sgm (Autodesk Fusion 360 design; units mm, degrees)
Autodesk Fusion 360 part; units mm, degrees
(part 1 of 2)
sketch "Sketch3" plane through (0, 0, 0) normal (0, 1, 0) x (1, 0, 0)
  spline S0 degree 3 poles (81.8621, -52.3081) (79.4279, -54.4777) (76.4646, -57.15) (75.3004, -58.2613) knots 0 0 0 0 1 1 1 1
  spline S1 degree 3 poles (75.3004, -58.2613) (74.1098, -59.3725) (73.0779, -60.1927) (72.9721, -60.0869) knots 0 0 0 0 1 1 1 1
  spline S2 degree 3 poles (72.9721, -60.0869) (72.5223, -59.6635) (72.1783, -56.6208) (72.3106, -54.3454) knots 0 0 0 0 1 1 1 1
  spline S3 degree 3 poles (72.3106, -54.3454) (72.4958, -51.5673) (72.2313, -50.9323) (70.776, -50.6412) knots 0 0 0 0 1 1 1 1
  spline S4 degree 3 poles (70.776, -50.6412) (69.559, -50.4296) (68.7652, -50.9587) (67.8392, -52.5727) knots 0 0 0 0 1 1 1 1
  spline S5 degree 3 poles (67.8392, -52.5727) (67.4423, -53.2871) (65.9606, -55.7477) (64.5583, -58.076) knots 0 0 0 0 1 1 1 1
  spline S6 degree 3 poles (64.5583, -58.076) (60.6954, -64.3996) (60.3779, -64.9817) (60.034, -66.1194) knots 0 0 0 0 1 1 1 1
  spline S7 degree 3 poles (60.034, -66.1194) (59.6371, -67.4423) (60.0075, -67.9979) (61.2246, -67.9979) knots 0 0 0 0 1 1 1 1
  spline S8 degree 3 poles (61.2246, -67.9979) (62.3888, -67.9979) (63.0238, -67.2306) (64.0027, -64.7171) knots 0 0 0 0 1 1 1 1
  spline S9 degree 3 poles (64.0027, -64.7171) (64.6906, -62.9444) (67.019, -58.4465) (68.8446, -55.4302) knots 0 0 0 0 1 1 1 1
  line L0 (68.8446, -55.4302) -> (69.3208, -54.6365)
  line L1 (69.3208, -54.6365) -> (69.2944, -57.15)
  spline S10 degree 3 poles (69.2944, -57.15) (69.2944, -60.3779) (69.85, -62.8915) (70.776, -63.6852) knots 0 0 0 0 1 1 1 1
  spline S11 degree 3 poles (70.776, -63.6852) (71.4375, -64.2673) (71.5169, -64.2673) (72.2842, -63.8704) knots 0 0 0 0 1 1 1 1
  spline S12 degree 3 poles (72.2842, -63.8704) (72.734, -63.6323) (75.1946, -61.4892) (77.7346, -59.1079) knots 0 0 0 0 1 1 1 1
  spline S13 degree 3 poles (77.7346, -59.1079) (80.301, -56.7267) (82.4442, -54.8217) (82.4706, -54.8746) knots 0 0 0 0 1 1 1 1
  spline S14 degree 3 poles (82.4706, -54.8746) (82.5235, -54.901) (81.6769, -56.7796) (80.5921, -59.0285) knots 0 0 0 0 1 1 1 1
  spline S15 degree 3 poles (80.5921, -59.0285) (77.2848, -65.9342) (76.7556, -68.7652) (78.6077, -69.4002) knots 0 0 0 0 1 1 1 1
  spline S16 degree 3 poles (78.6077, -69.4002) (79.2163, -69.6119) (80.5921, -68.924) (81.1213, -68.1567) knots 0 0 0 0 1 1 1 1
  spline S17 degree 3 poles (81.1213, -68.1567) (81.5181, -67.5217) (81.5181, -67.4158) (81.1477, -66.9925) knots 0 0 0 0 1 1 1 1
  spline S18 degree 3 poles (81.1477, -66.9925) (80.7773, -66.5692) (80.7508, -66.3575) (81.0683, -65.1933) knots 0 0 0 0 1 1 1 1
  spline S19 degree 3 poles (81.0683, -65.1933) (81.5446, -63.3677) (82.2854, -61.4627) (83.7406, -58.2083) knots 0 0 0 0 1 1 1 1
  spline S20 degree 3 poles (83.7406, -58.2083) (84.4285, -56.7002) (85.2223, -54.7952) (85.5133, -53.975) knots 0 0 0 0 1 1 1 1
  spline S21 degree 3 poles (85.5133, -53.975) (85.8308, -53.1813) (86.4658, -51.8848) (86.9421, -51.1175) knots 0 0 0 0 1 1 1 1
  spline S22 degree 3 poles (86.9421, -51.1175) (87.4448, -50.3502) (87.8417, -49.6358) (87.8417, -49.5035) knots 0 0 0 0 1 1 1 1
  spline S23 degree 3 poles (87.8417, -49.5035) (87.8417, -49.2125) (86.9421, -48.4188) (86.5717, -48.4188) knots 0 0 0 0 1 1 1 1
  spline S24 degree 3 poles (86.5717, -48.4188) (86.4129, -48.4188) (84.2963, -50.165) (81.8621, -52.3081) knots 0 0 0 0 1 1 1 1
  spline S25 degree 3 poles (149.9658, -49.9269) (148.934, -51.0381) (146.6585, -54.7952) (145.124, -57.9967) knots 0 0 0 0 1 1 1 1
  spline S26 degree 3 poles (145.124, -57.9967) (143.6688, -61.0394) (142.8221, -61.9125) (139.356, -64.135) knots 0 0 0 0 1 1 1 1
  spline S27 degree 3 poles (139.356, -64.135) (137.2394, -65.5108) (135.9165, -65.9342) (135.3079, -65.5108) knots 0 0 0 0 1 1 1 1
  spline S28 degree 3 poles (135.3079, -65.5108) (134.8846, -65.1933) (134.8846, -65.0875) (135.3079, -63.7646) knots 0 0 0 0 1 1 1 1
  spline S29 degree 3 poles (135.3079, -63.7646) (136.0223, -61.5685) (137.9538, -57.8908) (140.3879, -54.0808) knots 0 0 0 0 1 1 1 1
  spline S30 degree 3 poles (140.3879, -54.0808) (141.605, -52.1494) (142.6104, -50.4031) (142.6104, -50.165) knots 0 0 0 0 1 1 1 1
  spline S31 degree 3 poles (142.6104, -50.165) (142.6104, -49.9004) (142.3723, -49.7417) (141.949, -49.7417) knots 0 0 0 0 1 1 1 1
  spline S32 degree 3 poles (141.949, -49.7417) (140.5996, -49.7417) (138.2448, -52.5463) (135.7842, -57.1235) knots 0 0 0 0 1 1 1 1
  spline S33 degree 3 poles (135.7842, -57.1235) (134.8317, -58.8698) (134.3819, -59.346) (131.7096, -61.4627) knots 0 0 0 0 1 1 1 1
  spline S34 degree 3 poles (131.7096, -61.4627) (126.8942, -65.2992) (124.169, -66.8602) (123.4546, -66.1458) knots 0 0 0 0 1 1 1 1
  spline S35 degree 3 poles (123.4546, -66.1458) (123.0842, -65.7754) (123.9838, -63.3677) (125.5713, -60.5102) knots 0 0 0 0 1 1 1 1
  spline S36 degree 3 poles (125.5713, -60.5102) (126.365, -59.0815) (127, -57.7056) (127, -57.4146) knots 0 0 0 0 1 1 1 1
  spline S37 degree 3 poles (127, -57.4146) (127, -56.5944) (126.1004, -56.5679) (123.9573, -57.2823) knots 0 0 0 0 1 1 1 1
  spline S38 degree 3 poles (123.9573, -57.2823) (121.1263, -58.2348) (119.4858, -58.1554) (118.3217, -56.9648) knots 0 0 0 0 1 1 1 1
  spline S39 degree 3 poles (118.3217, -56.9648) (117.3163, -55.9594) (115.8081, -57.0442) (113.7179, -60.2456) knots 0 0 0 0 1 1 1 1
  spline S40 degree 3 poles (113.7179, -60.2456) (112.7919, -61.6744) (111.5748, -63.5265) (111.0456, -64.3467) knots 0 0 0 0 1 1 1 1
  spline S41 degree 3 poles (111.0456, -64.3467) (110.49, -65.1933) (109.9344, -65.8813) (109.7756, -65.8813) knots 0 0 0 0 1 1 1 1
  spline S42 degree 3 poles (109.7756, -65.8813) (109.4581, -65.8813) (109.5904, -61.2246) (109.9608, -58.5787) knots 0 0 0 0 1 1 1 1
  spline S43 degree 3 poles (109.9608, -58.5787) (110.0931, -57.7321) (110.0138, -57.441) (109.6963, -57.3352) knots 0 0 0 0 1 1 1 1
  spline S44 degree 3 poles (109.6963, -57.3352) (108.8231, -56.9913) (107.9235, -57.8379) (104.7221, -61.8331) knots 0 0 0 0 1 1 1 1
  spline S45 degree 3 poles (104.7221, -61.8331) (101.6, -65.8019) (101.4677, -65.9077) (101.3883, -65.0875) knots 0 0 0 0 1 1 1 1
  spline S46 degree 3 poles (101.3883, -65.0875) (101.3354, -64.6113) (101.4942, -63.0238) (101.7588, -61.5421) knots 0 0 0 0 1 1 1 1
  spline S47 degree 3 poles (101.7588, -61.5421) (101.9969, -60.0869) (102.235, -58.4465) (102.235, -57.9438) knots 0 0 0 0 1 1 1 1
  spline S48 degree 3 poles (102.235, -57.9438) (102.2615, -57.0706) (102.2085, -57.0177) (101.2825, -56.9383) knots 0 0 0 0 1 1 1 1
  spline S49 degree 3 poles (101.2825, -56.9383) (100.4094, -56.859) (100.2242, -56.9648) (99.7479, -57.7321) knots 0 0 0 0 1 1 1 1
  spline S50 degree 3 poles (99.7479, -57.7321) (98.9806, -59.0021) (98.6896, -60.8277) (98.6102, -64.9817) knots 0 0 0 0 1 1 1 1
  spline S51 degree 3 poles (98.6102, -64.9817) (98.5573, -69.0033) (98.716, -69.5854) (99.9067, -69.5854) knots 0 0 0 0 1 1 1 1
  spline S52 degree 3 poles (99.9067, -69.5854) (100.8327, -69.5854) (102.1556, -68.2625) (104.8279, -64.7171) knots 0 0 0 0 1 1 1 1
  line L2 (104.8279, -64.7171) -> (107.2356, -61.5156)
  line L3 (107.2356, -61.5156) -> (107.0504, -63.6323)
  spline S53 degree 3 poles (107.0504, -63.6323) (106.6271, -68.6065) (108.1352, -70.3792) (110.7281, -67.9715) knots 0 0 0 0 1 1 1 1
  spline S54 degree 3 poles (110.7281, -67.9715) (111.3896, -67.3629) (112.5802, -65.8019) (113.4269, -64.4525) knots 0 0 0 0 1 1 1 1
  spline S55 degree 3 poles (113.4269, -64.4525) (114.2471, -63.1296) (115.3054, -61.5421) (115.8081, -60.9335) knots 0 0 0 0 1 1 1 1
  spline S56 degree 3 poles (115.8081, -60.9335) (116.6283, -59.9017) (116.7342, -59.8488) (117.5544, -60.0869) knots 0 0 0 0 1 1 1 1
  spline S57 degree 3 poles (117.5544, -60.0869) (118.8773, -60.4573) (120.2531, -60.3779) (121.7348, -59.8223) knots 0 0 0 0 1 1 1 1
  spline S58 degree 3 poles (121.7348, -59.8223) (122.5815, -59.4783) (123.0313, -59.4254) (122.9519, -59.6106) knots 0 0 0 0 1 1 1 1
  spline S59 degree 3 poles (122.9519, -59.6106) (122.8725, -59.7958) (122.264, -61.2246) (121.6025, -62.8121) knots 0 0 0 0 1 1 1 1
  spline S60 degree 3 poles (121.6025, -62.8121) (120.0415, -66.4633) (119.8827, -67.3629) (120.65, -68.3419) knots 0 0 0 0 1 1 1 1
  spline S61 degree 3 poles (120.65, -68.3419) (121.0998, -68.8975) (121.4438, -69.0563) (122.264, -69.0563) knots 0 0 0 0 1 1 1 1
  spline S62 degree 3 poles (122.264, -69.0563) (124.2483, -69.0563) (127.4498, -67.3629) (131.0746, -64.3996) knots 0 0 0 0 1 1 1 1
  spline S63 degree 3 poles (131.0746, -64.3996) (131.8683, -63.7646) (132.5827, -63.2354) (132.6621, -63.2354) knots 0 0 0 0 1 1 1 1
  spline S64 degree 3 poles (132.6621, -63.2354) (132.7415, -63.2354) (132.6356, -63.7381) (132.424, -64.3202) knots 0 0 0 0 1 1 1 1
  spline S65 degree 3 poles (132.424, -64.3202) (131.4979, -66.9131) (132.1594, -68.3419) (134.2496, -68.3419) knots 0 0 0 0 1 1 1 1
  spline S66 degree 3 poles (134.2496, -68.3419) (135.7577, -68.3419) (137.8479, -67.3365) (140.626, -65.2198) knots 0 0 0 0 1 1 1 1
  line L4 (140.626, -65.2198) -> (142.7692, -63.6058)
  line L5 (142.7692, -63.6058) -> (142.531, -64.9817)
  spline S67 degree 3 poles (142.531, -64.9817) (142.1871, -66.9925) (142.7427, -68.1302) (144.2244, -68.5271) knots 0 0 0 0 1 1 1 1
  spline S68 degree 3 poles (144.2244, -68.5271) (146.05, -69.0298) (148.4577, -68.0508) (151.2888, -65.6696) knots 0 0 0 0 1 1 1 1
  spline S69 degree 3 poles (151.2888, -65.6696) (154.2256, -63.209) (154.1463, -61.9125) (151.1829, -64.0027) knots 0 0 0 0 1 1 1 1
  spline S70 degree 3 poles (151.1829, -64.0027) (149.225, -65.3785) (147.0819, -66.2517) (146.2881, -66.0135) knots 0 0 0 0 1 1 1 1
  spline S71 degree 3 poles (146.2881, -66.0135) (144.5419, -65.4579) (145.759, -61.8596) (150.9183, -52.361) knots 0 0 0 0 1 1 1 1
  spline S72 degree 3 poles (150.9183, -52.361) (151.6592, -50.9852) (152.0825, -49.9004) (151.9767, -49.6358) knots 0 0 0 0 1 1 1 1
  spline S73 degree 3 poles (151.9767, -49.6358) (151.7385, -48.9744) (150.7331, -49.1331) (149.9658, -49.9269) knots 0 0 0 0 1 1 1 1
  spline S74 degree 3 poles (56.9913, -49.8475) (51.0117, -51.1969) (44.0267, -56.4621) (41.5396, -61.4627) knots 0 0 0 0 1 1 1 1
  spline S75 degree 3 poles (41.5396, -61.4627) (39.8198, -64.9288) (40.0315, -66.7015) (42.254, -67.6275) knots 0 0 0 0 1 1 1 1
  spline S76 degree 3 poles (42.254, -67.6275) (43.8944, -68.3154) (46.3285, -67.9185) (50.0327, -66.3046) knots 0 0 0 0 1 1 1 1
  line L6 (50.0327, -66.3046) -> (52.0435, -65.4579)
  line L7 (52.0435, -65.4579) -> (50.7206, -67.6804)
  spline S77 degree 3 poles (50.7206, -67.6804) (49.5829, -69.6119) (49.4506, -69.9823) (49.7152, -70.5379) knots 0 0 0 0 1 1 1 1
  spline S78 degree 3 poles (49.7152, -70.5379) (49.9269, -71.0142) (50.1915, -71.1729) (50.8794, -71.1729) knots 0 0 0 0 1 1 1 1
  spline S79 degree 3 poles (50.8794, -71.1729) (52.0171, -71.1729) (52.4933, -70.6438) (53.5781, -68.1302) knots 0 0 0 0 1 1 1 1
  spline S80 degree 3 poles (53.5781, -68.1302) (54.5835, -65.8283) (56.1975, -63.0502) (57.5204, -61.304) knots 0 0 0 0 1 1 1 1
  spline S81 degree 3 poles (57.5204, -61.304) (59.3196, -58.9492) (59.399, -58.2083) (57.8379, -58.2083) knots 0 0 0 0 1 1 1 1
  spline S82 degree 3 poles (57.8379, -58.2083) (56.4621, -58.2083) (56.171, -58.3935) (55.1656, -60.0869) knots 0 0 0 0 1 1 1 1
  spline S83 degree 3 poles (55.1656, -60.0869) (54.1073, -61.8067) (53.4988, -62.3358) (50.8794, -63.6058) knots 0 0 0 0 1 1 1 1
  spline S84 degree 3 poles (50.8794, -63.6058) (47.7044, -65.1669) (44.741, -65.8019) (43.9738, -65.0346) knots 0 0 0 0 1 1 1 1
  spline S85 degree 3 poles (43.9738, -65.0346) (43.7885, -64.8494) (43.6563, -64.3731) (43.6563, -63.9763) knots 0 0 0 0 1 1 1 1
  spline S86 degree 3 poles (43.6563, -63.9763) (43.6563, -60.1398) (53.2871, -52.1229) (57.5204, -52.4404) knots 0 0 0 0 1 1 1 1
  spline S87 degree 3 poles (57.5204, -52.4404) (58.4994, -52.5198) (58.6052, -52.5992) (58.7375, -53.3135) knots 0 0 0 0 1 1 1 1
  spline S88 degree 3 poles (58.7375, -53.3135) (58.8433, -53.8692) (59.055, -54.1338) (59.4519, -54.1867) knots 0 0 0 0 1 1 1 1
  spline S89 degree 3 poles (59.4519, -54.1867) (60.2456, -54.2925) (62.4417, -52.1229) (62.4417, -51.1969) knots 0 0 0 0 1 1 1 1
  spline S90 degree 3 poles (62.4417, -51.1969) (62.4417, -49.7681) (60.0075, -49.186) (56.9913, -49.8475) knots 0 0 0 0 1 1 1 1
  spline S91 degree 3 poles (130.0427, -49.7681) (129.7252, -49.9269) (129.1431, -50.5883) (128.7463, -51.2762) knots 0 0 0 0 1 1 1 1
  spline S92 degree 3 poles (128.7463, -51.2762) (127.926, -52.6256) (128.0319, -53.2342) (129.1167, -53.3929) knots 0 0 0 0 1 1 1 1
  spline S93 degree 3 poles (129.1167, -53.3929) (129.7781, -53.4988) (131.2863, -52.2023) (131.9477, -50.9587) knots 0 0 0 0 1 1 1 1
  spline S94 degree 3 poles (131.9477, -50.9587) (132.3181, -50.2444) (132.3181, -50.1385) (131.8683, -49.821) knots 0 0 0 0 1 1 1 1
  spline S95 degree 3 poles (131.8683, -49.821) (131.3127, -49.4242) (130.7835, -49.3977) (130.0427, -49.7681) knots 0 0 0 0 1 1 1 1
  spline S96 degree 3 poles (34.6604, -51.0646) (30.4271, -51.9642) (27.6754, -53.4194) (26.7229, -55.2979) knots 0 0 0 0 1 1 1 1
  spline S97 degree 3 poles (26.7229, -55.2979) (26.0879, -56.5415) (26.0615, -56.9383) (26.6171, -58.1025) knots 0 0 0 0 1 1 1 1
  spline S98 degree 3 poles (26.6171, -58.1025) (27.1463, -59.2137) (28.7338, -60.2721) (31.5648, -61.4098) knots 0 0 0 0 1 1 1 1
  spline S99 degree 3 poles (31.5648, -61.4098) (33.999, -62.3623) (35.1896, -63.1031) (35.1896, -63.6323) knots 0 0 0 0 1 1 1 1
  spline S100 degree 3 poles (35.1896, -63.6323) (35.1896, -64.2144) (33.4433, -65.5373) (31.8294, -66.1458) knots 0 0 0 0 1 1 1 1
  spline S101 degree 3 poles (31.8294, -66.1458) (30.1625, -66.8073) (27.305, -66.966) (24.5798, -66.5692) knots 0 0 0 0 1 1 1 1
  spline S102 degree 3 poles (24.5798, -66.5692) (22.7277, -66.2781) (21.881, -66.6485) (22.0133, -67.6804) knots 0 0 0 0 1 1 1 1
  spline S103 degree 3 poles (22.0133, -67.6804) (22.1192, -68.6858) (23.0717, -69.0298) (25.9821, -69.215) knots 0 0 0 0 1 1 1 1
  spline S104 degree 3 poles (25.9821, -69.215) (30.1096, -69.4796) (33.7344, -68.3419) (36.2744, -65.9871) knots 0 0 0 0 1 1 1 1
  spline S105 degree 3 poles (36.2744, -65.9871) (38.6821, -63.7117) (38.9467, -62.4417) (37.3856, -60.8542) knots 0 0 0 0 1 1 1 1
  spline S106 degree 3 poles (37.3856, -60.8542) (36.6448, -60.1398) (35.7981, -59.69) (34.2635, -59.1608) knots 0 0 0 0 1 1 1 1
  spline S107 degree 3 poles (34.2635, -59.1608) (31.8029, -58.3406) (30.2419, -57.494) (29.7127, -56.7267) knots 0 0 0 0 1 1 1 1
  spline S108 degree 3 poles (29.7127, -56.7267) (29.3952, -56.2504) (29.4217, -56.0917) (29.9244, -55.4567) knots 0 0 0 0 1 1 1 1
  spline S109 degree 3 poles (29.9244, -55.4567) (30.2419, -55.0333) (31.0356, -54.4777) (31.6971, -54.2131) knots 0 0 0 0 1 1 1 1
  spline S110 degree 3 poles (31.6971, -54.2131) (33.2846, -53.5252) (37.2004, -52.8637) (38.444, -53.0754) knots 0 0 0 0 1 1 1 1
  spline S111 degree 3 poles (38.444, -53.0754) (39.4229, -53.2342) (39.4229, -53.2606) (39.2642, -54.1338) knots 0 0 0 0 1 1 1 1
  spline S112 degree 3 poles (39.2642, -54.1338) (39.1848, -54.6365) (39.2113, -55.0333) (39.3171, -55.0333) knots 0 0 0 0 1 1 1 1
  spline S113 degree 3 poles (39.3171, -55.0333) (39.7933, -55.0333) (41.275, -53.975) (41.6719, -53.34) knots 0 0 0 0 1 1 1 1
  spline S114 degree 3 poles (41.6719, -53.34) (43.2329, -50.9852) (39.9785, -49.9269) (34.6604, -51.0646) knots 0 0 0 0 1 1 1 1
  spline S115 degree 3 poles (169.9419, -51.3821) (167.984, -53.4194) (163.5919, -61.6744) (162.2954, -65.749) knots 0 0 0 0 1 1 1 1
  spline S116 degree 3 poles (162.2954, -65.749) (161.634, -67.8656) (161.6075, -69.506) (162.2425, -70.2998) knots 0 0 0 0 1 1 1 1
  spline S117 degree 3 poles (162.2425, -70.2998) (162.5865, -70.7496) (164.2004, -70.7231) (165.3646, -70.2733) knots 0 0 0 0 1 1 1 1
  spline S118 degree 3 poles (165.3646, -70.2733) (168.1427, -69.1885) (175.2865, -66.0929) (176.9004, -65.2727) knots 0 0 0 0 1 1 1 1
  line L8 (176.9004, -65.2727) -> (178.8054, -64.3202)
  line L9 (178.8054, -64.3202) -> (178.9642, -65.3521)
  spline S119 degree 3 poles (178.9642, -65.3521) (179.2288, -66.9925) (180.1548, -67.5481) (182.4567, -67.4158) knots 0 0 0 0 1 1 1 1
  spline S120 degree 3 poles (182.4567, -67.4158) (184.0442, -67.3365) (184.7056, -67.1512) (186.6635, -66.1723) knots 0 0 0 0 1 1 1 1
  spline S121 degree 3 poles (186.6635, -66.1723) (189.0713, -64.9817) (191.8229, -62.6798) (191.8229, -61.8331) knots 0 0 0 0 1 1 1 1
  spline S122 degree 3 poles (191.8229, -61.8331) (191.8229, -61.1188) (191.2938, -61.304) (189.1771, -62.7063) knots 0 0 0 0 1 1 1 1
  spline S123 degree 3 poles (189.1771, -62.7063) (187.3515, -63.9498) (184.5204, -65.0875) (183.3298, -65.0875) knots 0 0 0 0 1 1 1 1
  spline S124 degree 3 poles (183.3298, -65.0875) (182.6419, -65.0875) (181.7423, -64.135) (181.9275, -63.6323) knots 0 0 0 0 1 1 1 1
  spline S125 degree 3 poles (181.9275, -63.6323) (182.0333, -63.3942) (182.8271, -62.8385) (183.7267, -62.3887) knots 0 0 0 0 1 1 1 1
  spline S126 degree 3 poles (183.7267, -62.3887) (188.5685, -59.981) (191.3996, -56.4885) (189.8121, -54.9275) knots 0 0 0 0 1 1 1 1
  spline S127 degree 3 poles (189.8121, -54.9275) (189.1771, -54.266) (187.2456, -54.3983) (185.6581, -55.1921) knots 0 0 0 0 1 1 1 1
  spline S128 degree 3 poles (185.6581, -55.1921) (183.9383, -56.0917) (181.3454, -58.6581) (180.1548, -60.7219) knots 0 0 0 0 1 1 1 1
  spline S129 degree 3 poles (180.1548, -60.7219) (179.2288, -62.3094) (179.2023, -62.3094) (176.1067, -63.7117) knots 0 0 0 0 1 1 1 1
  spline S130 degree 3 poles (176.1067, -63.7117) (174.3604, -64.479) (172.9052, -65.061) (172.8523, -64.9817) knots 0 0 0 0 1 1 1 1
  spline S131 degree 3 poles (172.8523, -64.9817) (172.7994, -64.9288) (173.355, -64.1879) (174.1223, -63.3413) knots 0 0 0 0 1 1 1 1
  spline S132 degree 3 poles (174.1223, -63.3413) (176.2919, -60.8542) (176.6888, -59.4519) (175.551, -58.3142) knots 0 0 0 0 1 1 1 1
  spline S133 degree 3 poles (175.551, -58.3142) (175.0483, -57.8115) (174.7308, -57.7056) (174.1752, -57.8379) knots 0 0 0 0 1 1 1 1
  spline S134 degree 3 poles (174.1752, -57.8379) (172.7465, -58.1554) (170.2329, -59.4519) (168.5131, -60.7748) knots 0 0 0 0 1 1 1 1
  spline S135 degree 3 poles (168.5131, -60.7748) (167.5342, -61.5156) (166.6081, -62.1771) (166.4494, -62.3094) knots 0 0 0 0 1 1 1 1
  spline S136 degree 3 poles (166.4494, -62.3094) (165.9731, -62.574) (167.005, -60.6425) (168.9894, -57.494) knots 0 0 0 0 1 1 1 1
  spline S137 degree 3 poles (168.9894, -57.494) (172.3231, -52.1494) (172.8258, -50.7471) (171.45, -50.5883) knots 0 0 0 0 1 1 1 1
  spline S138 degree 3 poles (171.45, -50.5883) (170.9738, -50.5354) (170.524, -50.7735) (169.9419, -51.3821) knots 0 0 0 0 1 1 1 1
  spline S139 degree 3 poles (187.0604, -57.8908) (186.69, -58.5258) (183.0917, -61.1981) (182.88, -60.9865) knots 0 0 0 0 1 1 1 1
  spline S140 degree 3 poles (182.88, -60.9865) (182.7213, -60.8277) (184.0706, -58.8962) (184.9702, -57.9702) knots 0 0 0 0 1 1 1 1
  spline S141 degree 3 poles (184.9702, -57.9702) (186.5048, -56.4356) (187.8806, -56.3827) (187.0604, -57.8908) knots 0 0 0 0 1 1 1 1
  spline S142 degree 3 poles (173.3021, -60.6954) (173.3021, -61.8596) (168.4338, -66.5956) (166.026, -67.7598) knots 0 0 0 0 1 1 1 1
  spline S143 degree 3 poles (166.026, -67.7598) (163.5919, -68.924) (163.3008, -68.7917) (164.465, -67.0454) knots 0 0 0 0 1 1 1 1
  spline S144 degree 3 poles (164.465, -67.0454) (165.8144, -65.0081) (168.4602, -62.7063) (171.1854, -61.1452) knots 0 0 0 0 1 1 1 1
  spline S145 degree 3 poles (171.1854, -61.1452) (172.7994, -60.2456) (173.3021, -60.1398) (173.3021, -60.6954) knots 0 0 0 0 1 1 1 1
  spline S146 degree 3 poles (72.4694, -86.8892) (71.9402, -87.2596) (71.3846, -87.8681) (71.2258, -88.2915) knots 0 0 0 0 1 1 1 1
  spline S147 degree 3 poles (71.2258, -88.2915) (71.0671, -88.6883) (70.5644, -90.0113) (70.1146, -91.2019) knots 0 0 0 0 1 1 1 1
  spline S148 degree 3 poles (70.1146, -91.2019) (69.2415, -93.5038) (67.5481, -95.6998) (65.9606, -96.6258) knots 0 0 0 0 1 1 1 1
  line L10 (65.9606, -96.6258) -> (65.1933, -97.0756)
  line L11 (65.1933, -97.0756) -> (65.2992, -96.3348)
  spline S149 degree 3 poles (65.2992, -96.3348) (65.4579, -95.1706) (64.9552, -94.4827) (63.7646, -94.2975) knots 0 0 0 0 1 1 1 1
  spline S150 degree 3 poles (63.7646, -94.2975) (62.6004, -94.1123) (62.574, -94.0329) (62.9973, -92.6042) knots 0 0 0 0 1 1 1 1
  spline S151 degree 3 poles (62.9973, -92.6042) (63.3942, -91.2548) (63.1296, -90.2758) (62.2565, -89.9319) knots 0 0 0 0 1 1 1 1
  spline S152 degree 3 poles (62.2565, -89.9319) (60.7748, -89.3763) (58.7375, -90.805) (57.9438, -92.9481) knots 0 0 0 0 1 1 1 1
  spline S153 degree 3 poles (57.9438, -92.9481) (57.5733, -93.9535) (57.441, -94.0594) (56.3827, -94.2446) knots 0 0 0 0 1 1 1 1
  spline S154 degree 3 poles (56.3827, -94.2446) (54.4777, -94.5621) (53.3665, -95.5675) (53.0225, -97.2608) knots 0 0 0 0 1 1 1 1
  spline S155 degree 3 poles (53.0225, -97.2608) (52.8373, -98.2927) (53.684, -99.2188) (54.8217, -99.2188) knots 0 0 0 0 1 1 1 1
  spline S156 degree 3 poles (54.8217, -99.2188) (55.5625, -99.2188) (55.6154, -99.2717) (55.4567, -99.9331) knots 0 0 0 0 1 1 1 1
  spline S157 degree 3 poles (55.4567, -99.9331) (54.954, -102.1292) (54.954, -102.579) (55.536, -103.161) knots 0 0 0 0 1 1 1 1
  spline S158 degree 3 poles (55.536, -103.161) (56.1975, -103.8225) (56.9913, -103.8754) (58.0496, -103.3198) knots 0 0 0 0 1 1 1 1
  spline S159 degree 3 poles (58.0496, -103.3198) (59.0285, -102.7906) (59.0815, -102.8171) (58.8433, -103.505) knots 0 0 0 0 1 1 1 1
  spline S160 degree 3 poles (58.8433, -103.505) (58.5523, -104.5104) (57.9173, -105.0396) (56.9913, -105.0396) knots 0 0 0 0 1 1 1 1
  spline S161 degree 3 poles (56.9913, -105.0396) (55.9594, -105.0396) (54.4777, -106.2038) (53.975, -107.3944) knots 0 0 0 0 1 1 1 1
  spline S162 degree 3 poles (53.975, -107.3944) (53.5252, -108.5056) (54.0808, -109.6433) (55.1656, -109.7492) knots 0 0 0 0 1 1 1 1
  spline S163 degree 3 poles (55.1656, -109.7492) (56.3298, -109.8815) (56.4621, -110.146) (56.0917, -111.6277) knots 0 0 0 0 1 1 1 1
  spline S164 degree 3 poles (56.0917, -111.6277) (55.8271, -112.7919) (55.8271, -113.0829) (56.1975, -113.6385) knots 0 0 0 0 1 1 1 1
  spline S165 degree 3 poles (56.1975, -113.6385) (56.8854, -114.6969) (58.4465, -114.5646) (59.7694, -113.3475) knots 0 0 0 0 1 1 1 1
  spline S166 degree 3 poles (59.7694, -113.3475) (60.3515, -112.8448) (60.96, -111.9717) (61.1452, -111.4425) knots 0 0 0 0 1 1 1 1
  spline S167 degree 3 poles (61.1452, -111.4425) (61.5421, -110.1725) (61.6479, -110.0667) (62.8385, -109.8021) knots 0 0 0 0 1 1 1 1
  spline S168 degree 3 poles (62.8385, -109.8021) (63.6852, -109.6169) (63.791, -109.6433) (63.6852, -110.0138) knots 0 0 0 0 1 1 1 1
  spline S169 degree 3 poles (63.6852, -110.0138) (62.865, -112.8448) (62.865, -112.8977) (63.3148, -113.6121) knots 0 0 0 0 1 1 1 1
  spline S170 degree 3 poles (63.3148, -113.6121) (63.6852, -114.1677) (63.9763, -114.3) (64.8229, -114.3) knots 0 0 0 0 1 1 1 1
  spline S171 degree 3 poles (64.8229, -114.3) (66.4898, -114.3) (67.7069, -113.03) (68.6329, -110.2783) knots 0 0 0 0 1 1 1 1
  spline S172 degree 3 poles (68.6329, -110.2783) (70.2469, -105.5688) (72.6017, -103.4256) (76.9144, -102.7906) knots 0 0 0 0 1 1 1 1
  spline S173 degree 3 poles (76.9144, -102.7906) (79.031, -102.4731) (79.2956, -102.3673) (80.0894, -101.4942) knots 0 0 0 0 1 1 1 1
  spline S174 degree 3 poles (80.0894, -101.4942) (81.0419, -100.4623) (81.28, -99.0335) (80.5656, -98.3456) knots 0 0 0 0 1 1 1 1
  spline S175 degree 3 poles (80.5656, -98.3456) (80.354, -98.134) (79.4279, -97.8694) (78.5283, -97.7635) knots 0 0 0 0 1 1 1 1
  spline S176 degree 3 poles (78.5283, -97.7635) (76.6233, -97.5519) (75.6444, -96.9698) (75.0358, -95.6733) knots 0 0 0 0 1 1 1 1
  spline S177 degree 3 poles (75.0358, -95.6733) (74.4273, -94.3769) (74.5067, -93.001) (75.4063, -90.3552) knots 0 0 0 0 1 1 1 1
  spline S178 degree 3 poles (75.4063, -90.3552) (75.8825, -88.9529) (76.1206, -87.7888) (76.0413, -87.3919) knots 0 0 0 0 1 1 1 1
  spline S179 degree 3 poles (76.0413, -87.3919) (75.7238, -86.1219) (73.9775, -85.8838) (72.4694, -86.8892) knots 0 0 0 0 1 1 1 1
  spline S180 degree 3 poles (74.0833, -88.5825) (74.0833, -88.8471) (73.7923, -89.9319) (73.4219, -90.9638) knots 0 0 0 0 1 1 1 1
  spline S181 degree 3 poles (73.4219, -90.9638) (72.3635, -93.9535) (72.5752, -96.3348) (74.0569, -98.0017) knots 0 0 0 0 1 1 1 1
  spline S182 degree 3 poles (74.0569, -98.0017) (74.7183, -98.7425) (76.3323, -99.4833) (77.3642, -99.4833) knots 0 0 0 0 1 1 1 1
  spline S183 degree 3 poles (77.3642, -99.4833) (78.5283, -99.4833) (79.1104, -99.7215) (79.1104, -100.1713) knots 0 0 0 0 1 1 1 1
  spline S184 degree 3 poles (79.1104, -100.1713) (79.1104, -100.7004) (78.2373, -101.0708) (76.9408, -101.0708) knots 0 0 0 0 1 1 1 1
  spline S185 degree 3 poles (76.9408, -101.0708) (74.4008, -101.0973) (70.7496, -103.3198) (68.8446, -106.045) knots 0 0 0 0 1 1 1 1
  spline S186 degree 3 poles (68.8446, -106.045) (68.2625, -106.8652) (67.4688, -108.5056) (67.0719, -109.6698) knots 0 0 0 0 1 1 1 1
  spline S187 degree 3 poles (67.0719, -109.6698) (66.6485, -110.834) (66.1988, -111.9452) (66.0665, -112.104) knots 0 0 0 0 1 1 1 1
  spline S188 degree 3 poles (66.0665, -112.104) (65.7225, -112.5802) (64.7171, -112.5538) (64.9023, -112.104) knots 0 0 0 0 1 1 1 1
  spline S189 degree 3 poles (64.9023, -112.104) (65.6167, -110.199) (66.4104, -107.1827) (66.4104, -106.2831) knots 0 0 0 0 1 1 1 1
  spline S190 degree 3 poles (66.4104, -106.2831) (66.384, -104.2458) (64.9288, -102.0233) (63.156, -101.3619) knots 0 0 0 0 1 1 1 1
  spline S191 degree 3 poles (63.156, -101.3619) (62.7327, -101.2031) (61.939, -101.0708) (61.3569, -101.0708) knots 0 0 0 0 1 1 1 1
  spline S192 degree 3 poles (61.3569, -101.0708) (60.6425, -101.0708) (60.2456, -100.9385) (60.1398, -100.6475) knots 0 0 0 0 1 1 1 1
  spline S193 degree 3 poles (60.1398, -100.6475) (59.9017, -99.986) (60.4044, -99.7215) (62.2565, -99.4833) knots 0 0 0 0 1 1 1 1
  spline S194 degree 3 poles (62.2565, -99.4833) (64.6113, -99.1923) (66.4898, -98.2662) (68.4742, -96.4406) knots 0 0 0 0 1 1 1 1
  spline S195 degree 3 poles (68.4742, -96.4406) (70.4056, -94.6679) (71.1994, -93.4244) (72.099, -90.7521) knots 0 0 0 0 1 1 1 1
  spline S196 degree 3 poles (72.099, -90.7521) (72.4694, -89.6938) (72.8927, -88.6619) (73.0515, -88.4767) knots 0 0 0 0 1 1 1 1
  spline S197 degree 3 poles (73.0515, -88.4767) (73.4748, -87.9475) (74.0833, -88.0269) (74.0833, -88.5825) knots 0 0 0 0 1 1 1 1
  spline S198 degree 3 poles (61.1981, -92.2338) (61.1717, -92.4983) (61.0658, -93.2392) (60.96, -93.8742) knots 0 0 0 0 1 1 1 1
  spline S199 degree 3 poles (60.96, -93.8742) (60.7483, -95.2235) (61.304, -96.0438) (62.4681, -96.0438) knots 0 0 0 0 1 1 1 1
  spline S200 degree 3 poles (62.4681, -96.0438) (62.865, -96.0438) (63.2883, -96.176) (63.3677, -96.3083) knots 0 0 0 0 1 1 1 1
  spline S201 degree 3 poles (63.3677, -96.3083) (63.6588, -96.7846) (62.9444, -97.3667) (62.1242, -97.3667) knots 0 0 0 0 1 1 1 1
  spline S202 degree 3 poles (62.1242, -97.3667) (60.5631, -97.3667) (59.1873, -98.4779) (58.6052, -100.3035) knots 0 0 0 0 1 1 1 1
  spline S203 degree 3 poles (58.6052, -100.3035) (58.1819, -101.5206) (57.5469, -102.1027) (57.0971, -101.6529) knots 0 0 0 0 1 1 1 1
  spline S204 degree 3 poles (57.0971, -101.6529) (56.9648, -101.5206) (57.0442, -100.9121) (57.2823, -100.2771) knots 0 0 0 0 1 1 1 1
  spline S205 degree 3 poles (57.2823, -100.2771) (57.8908, -98.5573) (57.2823, -97.3667) (55.8006, -97.3667) knots 0 0 0 0 1 1 1 1
  spline S206 degree 3 poles (55.8006, -97.3667) (55.2185, -97.3667) (55.0333, -97.2344) (55.0333, -96.864) knots 0 0 0 0 1 1 1 1
  spline S207 degree 3 poles (55.0333, -96.864) (55.0333, -96.3348) (55.2979, -96.2025) (56.9119, -95.9379) knots 0 0 0 0 1 1 1 1
  spline S208 degree 3 poles (56.9119, -95.9379) (58.0231, -95.7527) (59.055, -94.7473) (59.69, -93.2656) knots 0 0 0 0 1 1 1 1
  spline S209 degree 3 poles (59.69, -93.2656) (59.9281, -92.6835) (60.2456, -92.0485) (60.4044, -91.8633) knots 0 0 0 0 1 1 1 1
  spline S210 degree 3 poles (60.4044, -91.8633) (60.7748, -91.4135) (61.251, -91.6252) (61.1981, -92.2338) knots 0 0 0 0 1 1 1 1
  spline S211 degree 3 poles (62.0713, -102.9758) (61.3304, -105.4629) (61.6744, -106.5477) (63.2354, -106.7858) knots 0 0 0 0 1 1 1 1
  spline S212 degree 3 poles (63.2354, -106.7858) (64.8229, -107.0504) (64.5054, -107.7119) (62.6269, -108.0558) knots 0 0 0 0 1 1 1 1
  spline S213 degree 3 poles (62.6269, -108.0558) (61.3304, -108.294) (59.8752, -109.5904) (59.5048, -110.8869) knots 0 0 0 0 1 1 1 1
  spline S214 degree 3 poles (59.5048, -110.8869) (59.1344, -112.051) (58.6581, -112.5802) (58.1025, -112.3685) knots 0 0 0 0 1 1 1 1
  spline S215 degree 3 poles (58.1025, -112.3685) (57.7585, -112.2363) (57.785, -112.0246) (58.129, -110.8869) knots 0 0 0 0 1 1 1 1
  spline S216 degree 3 poles (58.129, -110.8869) (58.5258, -109.6698) (58.5258, -109.5375) (58.129, -108.9025) knots 0 0 0 0 1 1 1 1
  spline S217 degree 3 poles (58.129, -108.9025) (57.8379, -108.4792) (57.3352, -108.1617) (56.7531, -108.0558) knots 0 0 0 0 1 1 1 1
  spline S218 degree 3 poles (56.7531, -108.0558) (55.4038, -107.8177) (55.6154, -107.1033) (57.15, -106.8123) knots 0 0 0 0 1 1 1 1
  spline S219 degree 3 poles (57.15, -106.8123) (59.1608, -106.4154) (60.034, -105.5158) (60.9335, -102.8435) knots 0 0 0 0 1 1 1 1
  spline S220 degree 3 poles (60.9335, -102.8435) (61.0394, -102.6054) (61.3569, -102.3938) (61.6744, -102.3938) knots 0 0 0 0 1 1 1 1
  spline S221 degree 3 poles (61.6744, -102.3938) (62.1242, -102.3938) (62.2035, -102.4996) (62.0713, -102.9758) knots 0 0 0 0 1 1 1 1
  spline S222 degree 3 poles (154.8077, -87.2067) (154.014, -87.8946) (153.6171, -88.5825) (153.1673, -89.9054) knots 0 0 0 0 1 1 1 1
  spline S223 degree 3 poles (153.1673, -89.9054) (152.056, -93.2921) (150.7596, -95.1971) (148.5371, -96.5994) knots 0 0 0 0 1 1 1 1
  line L12 (148.5371, -96.5994) -> (147.7433, -97.0756)
  line L13 (147.7433, -97.0756) -> (147.8492, -96.2025)
  spline S224 degree 3 poles (147.8492, -96.2025) (147.9815, -95.0648) (147.1877, -94.1917) (146.0235, -94.1917) knots 0 0 0 0 1 1 1 1
  spline S225 degree 3 poles (146.0235, -94.1917) (145.2563, -94.1917) (145.2033, -94.1388) (145.415, -93.4508) knots 0 0 0 0 1 1 1 1
  spline S226 degree 3 poles (145.415, -93.4508) (145.5208, -93.054) (145.6267, -92.2073) (145.6267, -91.5458) knots 0 0 0 0 1 1 1 1
  spline S227 degree 3 poles (145.6267, -91.5458) (145.6531, -90.514) (145.5738, -90.3288) (144.9123, -90.0113) knots 0 0 0 0 1 1 1 1
  spline S228 degree 3 poles (144.9123, -90.0113) (143.4306, -89.2969) (141.5785, -90.514) (140.5467, -92.8952) knots 0 0 0 0 1 1 1 1
  spline S229 degree 3 poles (140.5467, -92.8952) (140.0704, -94.0065) (139.9381, -94.1388) (138.9327, -94.271) knots 0 0 0 0 1 1 1 1
  spline S230 degree 3 poles (138.9327, -94.271) (137.504, -94.4563) (136.1281, -95.5146) (135.7313, -96.7317) knots 0 0 0 0 1 1 1 1
  spline S231 degree 3 poles (135.7313, -96.7317) (135.4402, -97.5783) (135.4667, -97.7635) (135.9165, -98.3985) knots 0 0 0 0 1 1 1 1
  spline S232 degree 3 poles (135.9165, -98.3985) (136.2604, -98.8219) (136.7367, -99.1129) (137.2658, -99.1658) knots 0 0 0 0 1 1 1 1
  spline S233 degree 3 poles (137.2658, -99.1658) (138.2183, -99.2717) (138.3242, -99.6156) (137.8215, -101.0444) knots 0 0 0 0 1 1 1 1
  spline S234 degree 3 poles (137.8215, -101.0444) (137.3981, -102.2085) (137.6892, -103.0552) (138.6417, -103.4521) knots 0 0 0 0 1 1 1 1
  spline S235 degree 3 poles (138.6417, -103.4521) (139.3296, -103.7431) (139.6206, -103.7167) (140.5202, -103.3727) knots 0 0 0 0 1 1 1 1
  spline S236 degree 3 poles (140.5202, -103.3727) (141.4727, -103.0023) (141.5785, -103.0023) (141.4463, -103.3463) knots 0 0 0 0 1 1 1 1
  spline S237 degree 3 poles (141.4463, -103.3463) (141.3669, -103.5844) (141.2875, -103.849) (141.2875, -103.9813) knots 0 0 0 0 1 1 1 1
  spline S238 degree 3 poles (141.2875, -103.9813) (141.2875, -104.5104) (140.3879, -105.0396) (139.5148, -105.0396) knots 0 0 0 0 1 1 1 1
  spline S239 degree 3 poles (139.5148, -105.0396) (138.774, -105.0396) (138.3506, -105.2513) (137.5569, -106.0715) knots 0 0 0 0 1 1 1 1
  spline S240 degree 3 poles (137.5569, -106.0715) (136.6838, -106.9181) (136.525, -107.2621) (136.525, -108.1617) knots 0 0 0 0 1 1 1 1
  spline S241 degree 3 poles (136.525, -108.1617) (136.525, -109.2994) (136.9748, -109.8021) (138.0331, -109.8021) knots 0 0 0 0 1 1 1 1
  spline S242 degree 3 poles (138.0331, -109.8021) (139.0385, -109.8021) (139.1973, -110.146) (138.774, -111.3631) knots 0 0 0 0 1 1 1 1
  spline S243 degree 3 poles (138.774, -111.3631) (138.2448, -112.8448) (138.2713, -113.1358) (138.9063, -113.7708) knots 0 0 0 0 1 1 1 1
  spline S244 degree 3 poles (138.9063, -113.7708) (140.0704, -114.935) (142.4252, -114.0619) (143.3777, -112.0775) knots 0 0 0 0 1 1 1 1
  spline S245 degree 3 poles (143.3777, -112.0775) (143.6952, -111.469) (143.9333, -110.834) (143.9333, -110.6488) knots 0 0 0 0 1 1 1 1
  spline S246 degree 3 poles (143.9333, -110.6488) (143.9333, -110.2519) (144.8065, -109.8021) (145.6267, -109.8021) knots 0 0 0 0 1 1 1 1
  spline S247 degree 3 poles (145.6267, -109.8021) (145.9971, -109.8021) (146.3146, -109.8285) (146.3146, -109.855) knots 0 0 0 0 1 1 1 1
  spline S248 degree 3 poles (146.3146, -109.855) (146.3146, -109.9079) (146.1294, -110.5165) (145.9177, -111.2308) knots 0 0 0 0 1 1 1 1
  spline S249 degree 3 poles (145.9177, -111.2308) (145.415, -112.9242) (145.415, -113.1358) (146.05, -113.7708) knots 0 0 0 0 1 1 1 1
  spline S250 degree 3 poles (146.05, -113.7708) (147.0554, -114.7763) (149.1456, -114.2471) (150.1775, -112.739) knots 0 0 0 0 1 1 1 1
  spline S251 degree 3 poles (150.1775, -112.739) (150.3892, -112.4479) (150.8654, -111.3631) (151.1829, -110.3842) knots 0 0 0 0 1 1 1 1
  spline S252 degree 3 poles (151.1829, -110.3842) (152.109, -107.6854) (152.744, -106.6006) (154.2256, -105.2248) knots 0 0 0 0 1 1 1 1
  spline S253 degree 3 poles (154.2256, -105.2248) (155.919, -103.6373) (157.3213, -103.0023) (159.6496, -102.7642) knots 0 0 0 0 1 1 1 1
  spline S254 degree 3 poles (159.6496, -102.7642) (161.0254, -102.6319) (161.634, -102.4202) (162.2425, -101.891) knots 0 0 0 0 1 1 1 1
  spline S255 degree 3 poles (162.2425, -101.891) (163.3008, -101.0179) (163.8565, -99.7215) (163.539, -98.8748) knots 0 0 0 0 1 1 1 1
  spline S256 degree 3 poles (163.539, -98.8748) (163.2479, -98.1075) (162.9569, -97.9752) (160.9196, -97.7371) knots 0 0 0 0 1 1 1 1
  spline S257 degree 3 poles (160.9196, -97.7371) (159.1469, -97.5519) (158.1415, -96.8375) (157.5329, -95.3558) knots 0 0 0 0 1 1 1 1
  spline S258 degree 3 poles (157.5329, -95.3558) (157.0038, -94.0594) (157.0831, -93.1598) (157.9563, -90.4081) knots 0 0 0 0 1 1 1 1
  spline S259 degree 3 poles (157.9563, -90.4081) (158.9088, -87.4712) (158.9088, -87.4712) (158.2208, -86.7833) knots 0 0 0 0 1 1 1 1
  spline S260 degree 3 poles (158.2208, -86.7833) (157.3742, -85.9367) (156.0248, -86.0954) (154.8077, -87.2067) knots 0 0 0 0 1 1 1 1
  spline S261 degree 3 poles (156.6863, -88.2385) (156.7656, -88.3179) (156.501, -89.4556) (156.0777, -90.7521) knots 0 0 0 0 1 1 1 1
  spline S262 degree 3 poles (156.0777, -90.7521) (155.1781, -93.5038) (155.1252, -95.1971) (155.8131, -96.7581) knots 0 0 0 0 1 1 1 1
  spline S263 degree 3 poles (155.8131, -96.7581) (156.4217, -98.0546) (157.9563, -99.1658) (159.4379, -99.3775) knots 0 0 0 0 1 1 1 1
  spline S264 degree 3 poles (159.4379, -99.3775) (161.29, -99.6421) (161.6604, -99.7479) (161.6604, -100.1448) knots 0 0 0 0 1 1 1 1
  spline S265 degree 3 poles (161.6604, -100.1448) (161.6604, -100.7004) (161.1577, -100.9121) (159.3585, -101.0973) knots 0 0 0 0 1 1 1 1
  spline S266 degree 3 poles (159.3585, -101.0973) (157.2154, -101.309) (155.1517, -102.3408) (153.1673, -104.1665) knots 0 0 0 0 1 1 1 1
  spline S267 degree 3 poles (153.1673, -104.1665) (151.3417, -105.8863) (150.6008, -107.0504) (149.5954, -109.8021) knots 0 0 0 0 1 1 1 1
  spline S268 degree 3 poles (149.5954, -109.8021) (148.8017, -112.0246) (148.4048, -112.5802) (147.7963, -112.3685) knots 0 0 0 0 1 1 1 1
  spline S269 degree 3 poles (147.7963, -112.3685) (147.4523, -112.2363) (147.5052, -111.8658) (148.1931, -109.8815) knots 0 0 0 0 1 1 1 1
  spline S270 degree 3 poles (148.1931, -109.8815) (149.9129, -104.9073) (148.4048, -101.5471) (144.2773, -101.0973) knots 0 0 0 0 1 1 1 1
  spline S271 degree 3 poles (144.2773, -101.0973) (143.1131, -100.965) (142.7163, -100.8327) (142.6633, -100.4888) knots 0 0 0 0 1 1 1 1
  spline S272 degree 3 poles (142.6633, -100.4888) (142.5575, -99.9067) (143.5365, -99.4833) (144.9388, -99.4833) knots 0 0 0 0 1 1 1 1
  spline S273 degree 3 poles (144.9388, -99.4833) (146.2881, -99.4569) (148.6958, -98.425) (150.4156, -97.1021) knots 0 0 0 0 1 1 1 1
  spline S274 degree 3 poles (150.4156, -97.1021) (152.2148, -95.6998) (153.6965, -93.5302) (154.649, -90.8315) knots 0 0 0 0 1 1 1 1
  spline S275 degree 3 poles (154.649, -90.8315) (155.0723, -89.6938) (155.5221, -88.609) (155.6544, -88.4238) knots 0 0 0 0 1 1 1 1
  spline S276 degree 3 poles (155.6544, -88.4238) (155.919, -88.1063) (156.4481, -88.0004) (156.6863, -88.2385) knots 0 0 0 0 1 1 1 1
  spline S277 degree 3 poles (143.7481, -92.2338) (143.7217, -92.4983) (143.6158, -93.2392) (143.51, -93.8742) knots 0 0 0 0 1 1 1 1
  spline S278 degree 3 poles (143.51, -93.8742) (143.2983, -95.2235) (143.854, -96.0438) (145.0181, -96.0438) knots 0 0 0 0 1 1 1 1
  spline S279 degree 3 poles (145.0181, -96.0438) (145.415, -96.0438) (145.8383, -96.176) (145.9177, -96.3083) knots 0 0 0 0 1 1 1 1
  spline S280 degree 3 poles (145.9177, -96.3083) (146.2088, -96.7846) (145.4944, -97.3667) (144.6213, -97.3667) knots 0 0 0 0 1 1 1 1
  spline S281 degree 3 poles (144.6213, -97.3667) (143.2983, -97.3667) (141.9754, -98.4515) (141.261, -100.1183) knots 0 0 0 0 1 1 1 1
  spline S282 degree 3 poles (141.261, -100.1183) (140.7054, -101.5206) (140.1763, -102.0233) (139.7, -101.7323) knots 0 0 0 0 1 1 1 1
  spline S283 degree 3 poles (139.7, -101.7323) (139.5677, -101.6529) (139.6471, -101.0973) (139.8588, -100.4888) knots 0 0 0 0 1 1 1 1
  spline S284 degree 3 poles (139.8588, -100.4888) (140.044, -99.9067) (140.2292, -99.1923) (140.2292, -98.9277) knots 0 0 0 0 1 1 1 1
  spline S285 degree 3 poles (140.2292, -98.9277) (140.2292, -98.1604) (139.2767, -97.3667) (138.3771, -97.3667) knots 0 0 0 0 1 1 1 1
  spline S286 degree 3 poles (138.3771, -97.3667) (137.9008, -97.3667) (137.5833, -97.2344) (137.5833, -97.0227) knots 0 0 0 0 1 1 1 1
  spline S287 degree 3 poles (137.5833, -97.0227) (137.5833, -96.4406) (138.1919, -96.0438) (139.0915, -96.0438) knots 0 0 0 0 1 1 1 1
  spline S288 degree 3 poles (139.0915, -96.0438) (140.1498, -96.0438) (141.9225, -94.5621) (142.2135, -93.4508) knots 0 0 0 0 1 1 1 1
  spline S289 degree 3 poles (142.2135, -93.4508) (142.584, -91.8898) (143.8804, -90.8579) (143.7481, -92.2338) knots 0 0 0 0 1 1 1 1
  spline S290 degree 3 poles (144.7271, -102.6848) (144.7271, -102.87) (144.5948, -103.4521) (144.436, -103.9813) knots 0 0 0 0 1 1 1 1
  spline S291 degree 3 poles (144.436, -103.9813) (143.9598, -105.5688) (144.2773, -106.2831) (145.6002, -106.6535) knots 0 0 0 0 1 1 1 1
  spline S292 degree 3 poles (145.6002, -106.6535) (146.976, -107.0504) (146.8967, -106.9975) (146.685, -107.5267) knots 0 0 0 0 1 1 1 1
  spline S293 degree 3 poles (146.685, -107.5267) (146.6056, -107.7648) (146.2352, -107.95) (145.9177, -107.95) knots 0 0 0 0 1 1 1 1
  spline S294 degree 3 poles (145.9177, -107.95) (144.3038, -107.95) (142.5575, -109.2465) (142.0548, -110.834) knots 0 0 0 0 1 1 1 1
  spline S295 degree 3 poles (142.0548, -110.834) (141.6844, -111.9981) (141.3404, -112.4479) (140.8377, -112.4479) knots 0 0 0 0 1 1 1 1
  spline S296 degree 3 poles (140.8377, -112.4479) (140.5202, -112.4479) (140.4673, -112.2627) (140.5996, -111.7071) knots 0 0 0 0 1 1 1 1
  spline S297 degree 3 poles (140.5996, -111.7071) (141.1023, -109.5375) (141.1023, -109.2465) (140.626, -108.7438) knots 0 0 0 0 1 1 1 1
  spline S298 degree 3 poles (140.626, -108.7438) (140.3615, -108.4527) (139.7529, -108.1617) (139.2502, -108.0558) knots 0 0 0 0 1 1 1 1
  spline S299 degree 3 poles (139.2502, -108.0558) (137.8744, -107.7913) (138.2183, -107.1298) (139.9117, -106.7594) knots 0 0 0 0 1 1 1 1
  spline S300 degree 3 poles (139.9117, -106.7594) (141.5785, -106.3625) (142.2665, -105.8069) (142.9544, -104.2458) knots 0 0 0 0 1 1 1 1
  spline S301 degree 3 poles (142.9544, -104.2458) (143.2454, -103.5844) (143.5894, -102.8965) (143.7217, -102.7113) knots 0 0 0 0 1 1 1 1
  spline S302 degree 3 poles (143.7217, -102.7113) (144.0656, -102.3144) (144.7271, -102.2879) (144.7271, -102.6848) knots 0 0 0 0 1 1 1 1
  spline S303 degree 3 poles (94.4298, -90.4875) (92.9217, -91.2812) (91.2283, -93.4244) (89.4292, -96.8375) knots 0 0 0 0 1 1 1 1
  spline S304 degree 3 poles (89.4292, -96.8375) (88.1592, -99.2717) (87.5506, -100.1448) (86.7569, -100.7004) knots 0 0 0 0 1 1 1 1
  spline S305 degree 3 poles (86.7569, -100.7004) (85.6456, -101.4677) (85.3546, -102.3938) (86.2277, -102.3938) knots 0 0 0 0 1 1 1 1
  spline S306 degree 3 poles (86.2277, -102.3938) (86.7304, -102.3938) (86.704, -102.4731) (86.069, -104.0342) knots 0 0 0 0 1 1 1 1
  spline S307 degree 3 poles (86.069, -104.0342) (84.8254, -107.1298) (82.5765, -111.2573) (81.6504, -112.1569) knots 0 0 0 0 1 1 1 1
  spline S308 degree 3 poles (81.6504, -112.1569) (80.8302, -112.9506) (80.6715, -113.0035) (79.9571, -112.7654) knots 0 0 0 0 1 1 1 1
  spline S309 degree 3 poles (79.9571, -112.7654) (78.449, -112.2363) (77.3642, -113.8767) (78.5283, -114.9085) knots 0 0 0 0 1 1 1 1
  spline S310 degree 3 poles (78.5283, -114.9085) (79.6131, -115.914) (81.8356, -115.0144) (83.8729, -112.8183) knots 0 0 0 0 1 1 1 1
  spline S311 degree 3 poles (83.8729, -112.8183) (85.1165, -111.4425) (86.995, -108.0029) (88.9794, -103.505) knots 0 0 0 0 1 1 1 1
  spline S312 degree 3 poles (88.9794, -103.505) (89.5615, -102.2085) (89.8525, -101.8646) (90.3023, -101.8646) knots 0 0 0 0 1 1 1 1
  spline S313 degree 3 poles (90.3023, -101.8646) (90.8579, -101.8646) (95.4352, -100.7533) (96.3877, -100.4094) knots 0 0 0 0 1 1 1 1
  spline S314 degree 3 poles (96.3877, -100.4094) (96.7317, -100.2506) (96.6258, -100.6475) (95.8585, -102.2615) knots 0 0 0 0 1 1 1 1
  spline S315 degree 3 poles (95.8585, -102.2615) (94.6944, -104.7221) (94.4033, -106.8388) (95.1177, -107.4208) knots 0 0 0 0 1 1 1 1
  spline S316 degree 3 poles (95.1177, -107.4208) (95.6998, -107.8971) (97.5254, -107.8971) (98.7425, -107.4208) knots 0 0 0 0 1 1 1 1
  spline S317 degree 3 poles (98.7425, -107.4208) (100.0919, -106.8652) (102.3938, -105.3571) (103.7167, -104.14) knots 0 0 0 0 1 1 1 1
  line L14 (103.7167, -104.14) -> (104.9073, -103.0552)
  line L15 (104.9073, -103.0552) -> (105.0396, -104.484)
  spline S318 degree 3 poles (105.0396, -104.484) (105.2248, -106.1244) (105.701, -106.6271) (107.1827, -106.6271) knots 0 0 0 0 1 1 1 1
  spline S319 degree 3 poles (107.1827, -106.6271) (108.4527, -106.6271) (110.9398, -105.3306) (113.1094, -103.5315) knots 0 0 0 0 1 1 1 1
  spline S320 degree 3 poles (113.1094, -103.5315) (114.0619, -102.7642) (114.8292, -102.1821) (114.8292, -102.2615) knots 0 0 0 0 1 1 1 1
  spline S321 degree 3 poles (114.8292, -102.2615) (114.8292, -102.3408) (114.3, -103.4785) (113.6385, -104.775) knots 0 0 0 0 1 1 1 1
  spline S322 degree 3 poles (113.6385, -104.775) (112.2892, -107.4473) (112.1833, -108.1352) (113.0565, -108.4527) knots 0 0 0 0 1 1 1 1
  spline S323 degree 3 poles (113.0565, -108.4527) (114.009, -108.8231) (114.7498, -108.3469) (117.6602, -105.5423) knots 0 0 0 0 1 1 1 1
  spline S324 degree 3 poles (117.6602, -105.5423) (121.4702, -101.9175) (121.3908, -101.944) (121.2321, -104.5104) knots 0 0 0 0 1 1 1 1
  spline S325 degree 3 poles (121.2321, -104.5104) (121.1263, -106.5477) (121.1263, -106.6271) (121.92, -107.4208) knots 0 0 0 0 1 1 1 1
  spline S326 degree 3 poles (121.92, -107.4208) (122.6344, -108.1352) (122.899, -108.2146) (124.3013, -108.2146) knots 0 0 0 0 1 1 1 1
  spline S327 degree 3 poles (124.3013, -108.2146) (126.1269, -108.2146) (127.291, -107.8706) (128.6404, -106.9181) knots 0 0 0 0 1 1 1 1
  spline S328 degree 3 poles (128.6404, -106.9181) (129.6194, -106.2038) (130.6248, -104.8544) (130.3338, -104.5898) knots 0 0 0 0 1 1 1 1
  spline S329 degree 3 poles (130.3338, -104.5898) (130.2544, -104.5104) (129.3548, -104.8015) (128.3758, -105.2513) knots 0 0 0 0 1 1 1 1
  spline S330 degree 3 poles (128.3758, -105.2513) (126.4179, -106.1773) (125.2802, -106.3096) (124.4865, -105.7275) knots 0 0 0 0 1 1 1 1
  spline S331 degree 3 poles (124.4865, -105.7275) (123.7456, -105.1983) (123.8515, -103.1875) (124.751, -100.9915) knots 0 0 0 0 1 1 1 1
  spline S332 degree 3 poles (124.751, -100.9915) (125.7829, -98.3721) (125.386, -97.8958) (123.0577, -98.9806) knots 0 0 0 0 1 1 1 1
  spline S333 degree 3 poles (123.0577, -98.9806) (121.7877, -99.5363) (120.4648, -100.5681) (117.9777, -102.87) knots 0 0 0 0 1 1 1 1
  spline S334 degree 3 poles (117.9777, -102.87) (117.1046, -103.6637) (116.4167, -104.2194) (116.4167, -104.1135) knots 0 0 0 0 1 1 1 1
  spline S335 degree 3 poles (116.4167, -104.1135) (116.4167, -104.0342) (117.131, -102.6848) (117.9777, -101.1238) knots 0 0 0 0 1 1 1 1
  spline S336 degree 3 poles (117.9777, -101.1238) (119.9885, -97.5254) (120.1208, -96.8375) (118.8244, -96.8375) knots 0 0 0 0 1 1 1 1
  spline S337 degree 3 poles (118.8244, -96.8375) (118.2158, -96.8375) (117.6602, -97.2079) (116.3638, -98.4779) knots 0 0 0 0 1 1 1 1
  spline S338 degree 3 poles (116.3638, -98.4779) (112.739, -102.0233) (109.1142, -104.484) (108.0823, -104.0871) knots 0 0 0 0 1 1 1 1
  spline S339 degree 3 poles (108.0823, -104.0871) (107.3679, -103.796) (107.7383, -102.1821) (109.1671, -99.2188) knots 0 0 0 0 1 1 1 1
  spline S340 degree 3 poles (109.1671, -99.2188) (110.4371, -96.5465) (110.5165, -95.7792) (109.511, -95.7792) knots 0 0 0 0 1 1 1 1
  spline S341 degree 3 poles (109.511, -95.7792) (108.876, -95.7792) (107.8971, -96.7846) (106.1508, -99.2188) knots 0 0 0 0 1 1 1 1
  spline S342 degree 3 poles (106.1508, -99.2188) (103.6373, -102.6848) (98.2927, -106.3096) (97.499, -105.0396) knots 0 0 0 0 1 1 1 1
  spline S343 degree 3 poles (97.499, -105.0396) (97.2873, -104.6956) (98.1604, -102.7377) (99.5098, -100.4888) knots 0 0 0 0 1 1 1 1
  spline S344 degree 3 poles (99.5098, -100.4888) (100.0919, -99.5098) (100.5417, -98.5044) (100.4888, -98.2398) knots 0 0 0 0 1 1 1 1
  spline S345 degree 3 poles (100.4888, -98.2398) (100.3829, -97.6048) (99.5363, -97.499) (98.5573, -97.9752) knots 0 0 0 0 1 1 1 1
  spline S346 degree 3 poles (98.5573, -97.9752) (97.2608, -98.6631) (90.7521, -99.8008) (90.7521, -99.351) knots 0 0 0 0 1 1 1 1
  spline S347 degree 3 poles (90.7521, -99.351) (90.7521, -98.9806) (92.4983, -95.7527) (93.4508, -94.2975) knots 0 0 0 0 1 1 1 1
  spline S348 degree 3 poles (93.4508, -94.2975) (95.4088, -91.3606) (96.4406, -91.5458) (95.0383, -94.5885) knots 0 0 0 0 1 1 1 1
  spline S349 degree 3 poles (95.0383, -94.5885) (94.5885, -95.5146) (94.324, -96.3613) (94.4563, -96.4406) knots 0 0 0 0 1 1 1 1
  spline S350 degree 3 poles (94.4563, -96.4406) (95.3294, -96.9963) (98.1604, -93.2127) (98.1604, -91.5194) knots 0 0 0 0 1 1 1 1
  spline S351 degree 3 poles (98.1604, -91.5194) (98.1604, -90.7785) (98.0281, -90.4346) (97.6577, -90.2229) knots 0 0 0 0 1 1 1 1
  spline S352 degree 3 poles (97.6577, -90.2229) (96.864, -89.826) (95.4881, -89.9319) (94.4298, -90.4875) knots 0 0 0 0 1 1 1 1
  line L16 (0, 0) -> (221.0158, 0)
  line L17 (221.0158, 0) -> (221.0158, -135.2462)
  line L18 (221.0158, -135.2462) -> (0, -135.2462)
  line L19 (0, -135.2462) -> (0, 0)
  constraint horizontal L16
  constraint vertical L17
  constraint horizontal L18
  constraint vertical L19
  constraint coincident L16.start L19.end